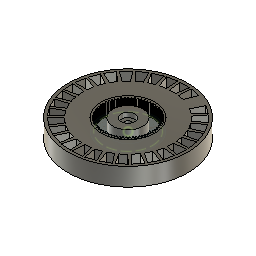
pillbox_disc2 v11 (Autodesk Fusion 360 design; units mm, degrees)
description: Internal Gear; Module: 1.270000; Number of Teeth: 64; Pressure Angle: 20.000000; Root Fillet Radius: 0.040000; Clearance: 0.000000; Gear Thickness: 2.000000; Outer Diameter: 10.000000;
Autodesk Fusion 360 part; units mm, degrees
(part 1 of 2)
sketch "Sketch1" plane through (0, 0, 0) normal (0, 0, 1) x (1, 0, 0)
  circle A0 centre (0, 0) radius 100
  dimension "d3" = 200
  constraint coincident A0.centre origin
  measures "d3" diameter of A0
extrude "Extrude1" add sketch "Sketch1" along normal blind 30 makes body 1
sketch "Sketch2" plane through (0, 0, 30) normal (0, 0, 1) x (-1, 0, 0)
  circle A0 centre (0, 0) radius 100
  line L0 (8, -95) -> (-8, -95)
  line L1 (-8, -95) -> (-5, -75)
  line L2 (-5, -75) -> (5, -75)
  line L3 (5, -75) -> (8, -95)
  line L4 (11.2871, -94.6657) -> (10.1997, -74.4712)
  line L5 (19.995, -72.4583) -> (26.9596, -91.445)
  line L6 (26.9596, -91.445) -> (11.2871, -94.6657)
  line L7 (10.1997, -74.4712) -> (19.995, -72.4583)
  line L8 (30.1121, -90.4558) -> (24.9819, -70.8936)
  line L9 (34.1715, -66.9501) -> (44.8155, -84.1461)
  line L10 (44.8155, -84.1461) -> (30.1121, -90.4558)
  line L11 (24.9819, -70.8936) -> (34.1715, -66.9501)
  line L12 (47.7044, -82.5427) -> (38.7413, -64.4136)
  line L13 (46.9489, -58.7009) -> (60.8366, -73.4024)
  line L14 (60.8366, -73.4024) -> (47.7044, -82.5427)
  line L15 (38.7413, -64.4136) -> (46.9489, -58.7009)
  line L16 (63.3436, -71.2502) -> (50.9146, -55.2965)
  line L17 (57.8043, -48.0486) -> (74.3671, -59.6535)
  line L18 (74.3671, -59.6535) -> (63.3436, -71.2502)
  line L19 (50.9146, -55.2965) -> (57.8043, -48.0486)
  line L20 (76.3895, -57.0407) -> (61.0035, -43.9155)
  line L21 (66.2931, -35.4291) -> (84.8529, -43.4624)
  line L22 (84.8529, -43.4624) -> (76.3895, -57.0407)
  line L23 (61.0035, -43.9155) -> (66.2931, -35.4291)
  line L24 (86.308, -40.496) -> (68.5949, -30.7367)
  line L25 (72.0679, -21.3591) -> (91.8649, -25.492)
  line L26 (91.8649, -25.492) -> (86.308, -40.496)
  line L27 (68.5949, -30.7367) -> (72.0679, -21.3591)
  line L28 (92.6931, -22.2934) -> (73.378, -16.2994)
  line L29 (74.8923, -6.4147) -> (95.1159, -6.4779)
  line L30 (95.1159, -6.4779) -> (92.6931, -22.2934)
  line L31 (73.378, -16.2994) -> (74.8923, -6.4147)
  line L32 (95.2833, -3.1781) -> (75.157, -1.1949)
  line L33 (74.6505, 8.7923) -> (94.4729, 12.8014)
  line L34 (94.4729, 12.8014) -> (95.2833, -3.1781)
  line L35 (75.157, -1.1949) -> (74.6505, 8.7923)
  line L36 (93.9725, 16.0674) -> (73.859, 13.9586)
  line L37 (71.3525, 23.6393) -> (89.9621, 31.5566)
  line L38 (89.9621, 31.5566) -> (93.9725, 16.0674)
  line L39 (73.859, 13.9586) -> (71.3525, 23.6393)
  line L40 (88.8146, 34.655) -> (69.5373, 28.5405)
  line L41 (65.1334, 37.5186) -> (81.7683, 49.0199)
  line L42 (81.7683, 49.0199) -> (88.8146, 34.655)
  line L43 (69.5373, 28.5405) -> (65.1334, 37.5186)
  line L44 (80.0205, 51.8239) -> (62.3687, 41.9541)
  line L45 (56.2477, 49.8618) -> (70.2268, 64.4763)
  line L46 (70.2268, 64.4763) -> (80.0205, 51.8239)
  line L47 (62.3687, 41.9541) -> (56.2477, 49.8618)
  line L48 (67.9505, 66.871) -> (52.6467, 53.65)
  line L49 (45.0591, 60.1637) -> (55.8103, 77.293)
  line L50 (55.8103, 77.293) -> (67.9505, 66.871)
  line L51 (52.6467, 53.65) -> (45.0591, 60.1637)
  line L52 (53.0985, 79.1805) -> (40.7694, 63.1495)
  line L53 (32.0259, 68.0025) -> (39.1089, 86.9453)
  line L54 (39.1089, 86.9453) -> (53.0985, 79.1805)
  line L55 (40.7694, 63.1495) -> (32.0259, 68.0025)
  line L56 (36.0726, 88.2483) -> (27.2229, 70.0636)
  line L57 (17.6815, 73.0573) -> (20.8064, 93.0381)
  line L58 (20.8064, 93.0381) -> (36.0726, 88.2483)
  line L59 (27.2229, 70.0636) -> (17.6815, 73.0573)
  line L60 (17.5699, 93.7032) -> (12.562, 74.1094)
  line L61 (2.6133, 75.121) -> (1.652, 95.3219)
  line L62 (1.652, 95.3219) -> (17.5699, 93.7032)
  line L63 (12.562, 74.1094) -> (2.6133, 75.121)
  line L64 (-1.652, 95.3219) -> (-2.6133, 75.121)
  line L65 (-12.562, 74.1094) -> (-17.5699, 93.7032)
  line L66 (-17.5699, 93.7032) -> (-1.652, 95.3219)
  line L67 (-2.6133, 75.121) -> (-12.562, 74.1094)
  line L68 (-20.8064, 93.0381) -> (-17.6815, 73.0573)
  line L69 (-27.2229, 70.0636) -> (-36.0726, 88.2483)
  line L70 (-36.0726, 88.2483) -> (-20.8064, 93.0381)
  line L71 (-17.6815, 73.0573) -> (-27.2229, 70.0636)
  line L72 (-39.1089, 86.9453) -> (-32.0259, 68.0025)
  line L73 (-40.7694, 63.1495) -> (-53.0985, 79.1805)
  line L74 (-53.0985, 79.1805) -> (-39.1089, 86.9453)
  line L75 (-32.0259, 68.0025) -> (-40.7694, 63.1495)
  line L76 (-55.8103, 77.293) -> (-45.0591, 60.1637)
  line L77 (-52.6467, 53.65) -> (-67.9505, 66.871)
  line L78 (-67.9505, 66.871) -> (-55.8103, 77.293)
  line L79 (-45.0591, 60.1637) -> (-52.6467, 53.65)
  line L80 (-70.2268, 64.4763) -> (-56.2477, 49.8618)
  line L81 (-62.3687, 41.9541) -> (-80.0205, 51.8239)
  line L82 (-80.0205, 51.8239) -> (-70.2268, 64.4763)
  line L83 (-56.2477, 49.8618) -> (-62.3687, 41.9541)
  line L84 (-81.7683, 49.0199) -> (-65.1334, 37.5186)
  line L85 (-69.5373, 28.5405) -> (-88.8146, 34.655)
  line L86 (-88.8146, 34.655) -> (-81.7683, 49.0199)
  line L87 (-65.1334, 37.5186) -> (-69.5373, 28.5405)
  line L88 (-89.9621, 31.5566) -> (-71.3525, 23.6393)
  line L89 (-73.859, 13.9586) -> (-93.9725, 16.0674)
  line L90 (-93.9725, 16.0674) -> (-89.9621, 31.5566)
  line L91 (-71.3525, 23.6393) -> (-73.859, 13.9586)
  line L92 (-94.4729, 12.8014) -> (-74.6505, 8.7923)
  line L93 (-75.157, -1.1949) -> (-95.2833, -3.1781)
  line L94 (-95.2833, -3.1781) -> (-94.4729, 12.8014)
  line L95 (-74.6505, 8.7923) -> (-75.157, -1.1949)
  line L96 (-95.1159, -6.4779) -> (-74.8923, -6.4147)
  line L97 (-73.378, -16.2994) -> (-92.6931, -22.2934)
  line L98 (-92.6931, -22.2934) -> (-95.1159, -6.4779)
  line L99 (-74.8923, -6.4147) -> (-73.378, -16.2994)
  line L100 (-91.8649, -25.492) -> (-72.0679, -21.3591)
  line L101 (-68.5949, -30.7367) -> (-86.308, -40.496)
  line L102 (-86.308, -40.496) -> (-91.8649, -25.492)
  line L103 (-72.0679, -21.3591) -> (-68.5949, -30.7367)
  line L104 (-84.8529, -43.4624) -> (-66.2931, -35.4291)
  line L105 (-61.0035, -43.9155) -> (-76.3895, -57.0407)
  line L106 (-76.3895, -57.0407) -> (-84.8529, -43.4624)
  line L107 (-66.2931, -35.4291) -> (-61.0035, -43.9155)
  line L108 (-74.3671, -59.6535) -> (-57.8043, -48.0486)
  line L109 (-50.9146, -55.2965) -> (-63.3436, -71.2502)
  line L110 (-63.3436, -71.2502) -> (-74.3671, -59.6535)
  line L111 (-57.8043, -48.0486) -> (-50.9146, -55.2965)
  line L112 (-60.8366, -73.4024) -> (-46.9489, -58.7009)
  line L113 (-38.7413, -64.4136) -> (-47.7044, -82.5427)
  line L114 (-47.7044, -82.5427) -> (-60.8366, -73.4024)
  line L115 (-46.9489, -58.7009) -> (-38.7413, -64.4136)
  line L116 (-44.8155, -84.1461) -> (-34.1715, -66.9501)
  line L117 (-24.9819, -70.8936) -> (-30.1121, -90.4558)
  line L118 (-30.1121, -90.4558) -> (-44.8155, -84.1461)
  line L119 (-34.1715, -66.9501) -> (-24.9819, -70.8936)
  line L120 (-26.9596, -91.445) -> (-19.995, -72.4583)
  line L121 (-10.1997, -74.4712) -> (-11.2871, -94.6657)
  line L122 (-11.2871, -94.6657) -> (-26.9596, -91.445)
  line L123 (-19.995, -72.4583) -> (-10.1997, -74.4712)
  dimension "d7" = 360
  constraint horizontal L0
  constraint parallel L0 L2
extrude "Extrude2" cut sketch "Sketch2" against normal blind 30 contours L0 L1 L2 L3 | L4 L5 L6 L7 | L8 L9 L10 L11 | L12 L13 L14 L15 | L16 L17 L18 L19 | L20 L21 L22 L23 | L24 L25 L26 L27 | L28 L29 L30 L31 | L32 L33 L34 L35 | L36 L37 L38 L39 | L40 L41 L42 L43 | L44 L45 L46 L47 | L48 L49 L50 L51 | L52 L53 L54 L55 | L56 L57 L58 L59 | L60 L61 L62 L63 | L64 L65 L66 L67 | L68 L69 L70 L71 | L72 L73 L74 L75 | L76 L77 L78 L79 | L80 L81 L82 L83 | L84 L85 L86 L87 | L88 L89 L90 L91 | L92 L93 L94 L95 | L96 L97 L98 L99 | L100 L101 L102 L103 | L104 L105 L106 L107 | L108 L109 L110 L111 | L112 L113 L114 L115 | L120 L121 L122 L123 bodies 1
sketch "Sketch3" plane through (0, 0, 30) normal (0, 0, 1) x (-1, 0, 0)
  line L0 (26.9596, -91.445) -> (11.2871, -94.6657)
  line L1 (11.2871, -94.6657) -> (10.1997, -74.4712)
  line L2 (10.1997, -74.4712) -> (19.995, -72.4583)
  line L3 (19.995, -72.4583) -> (26.9596, -91.445)
  line L4 (84.8529, -43.4624) -> (76.3895, -57.0407)
  line L5 (76.3895, -57.0407) -> (61.0035, -43.9155)
  line L6 (61.0035, -43.9155) -> (66.2931, -35.4291)
  line L7 (66.2931, -35.4291) -> (84.8529, -43.4624)
  line L8 (89.9621, 31.5566) -> (93.9725, 16.0674)
  line L9 (93.9725, 16.0674) -> (73.859, 13.9586)
  line L10 (73.859, 13.9586) -> (71.3525, 23.6393)
  line L11 (71.3525, 23.6393) -> (89.9621, 31.5566)
  line L12 (39.1089, 86.9453) -> (53.0985, 79.1805)
  line L13 (53.0985, 79.1805) -> (40.7694, 63.1495)
  line L14 (40.7694, 63.1495) -> (32.0259, 68.0025)
  line L15 (32.0259, 68.0025) -> (39.1089, 86.9453)
  line L16 (-36.0726, 88.2483) -> (-20.8064, 93.0381)
  line L17 (-20.8064, 93.0381) -> (-17.6815, 73.0573)
  line L18 (-17.6815, 73.0573) -> (-27.2229, 70.0636)
  line L19 (-27.2229, 70.0636) -> (-36.0726, 88.2483)
  line L20 (-88.8146, 34.655) -> (-81.7683, 49.0199)
  line L21 (-81.7683, 49.0199) -> (-65.1334, 37.5186)
  line L22 (-65.1334, 37.5186) -> (-69.5373, 28.5405)
  line L23 (-69.5373, 28.5405) -> (-88.8146, 34.655)
  line L24 (-86.308, -40.496) -> (-91.8649, -25.492)
  line L25 (-91.8649, -25.492) -> (-72.0679, -21.3591)
  line L26 (-72.0679, -21.3591) -> (-68.5949, -30.7367)
  line L27 (-68.5949, -30.7367) -> (-86.308, -40.496)
  line L28 (-47.7044, -82.5427) -> (-60.8366, -73.4024)
  line L29 (-60.8366, -73.4024) -> (-46.9489, -58.7009)
  line L30 (-46.9489, -58.7009) -> (-38.7413, -64.4136)
  line L31 (-38.7413, -64.4136) -> (-47.7044, -82.5427)
  line L32 (-92.6931, -22.2934) -> (-95.1159, -6.4779)
  line L33 (-95.1159, -6.4779) -> (-74.8923, -6.4147)
  line L34 (-74.8923, -6.4147) -> (-73.378, -16.2994)
  line L35 (-73.378, -16.2994) -> (-92.6931, -22.2934)
  line L36 (-80.0205, 51.8239) -> (-70.2268, 64.4763)
  line L37 (-70.2268, 64.4763) -> (-56.2477, 49.8618)
  line L38 (-56.2477, 49.8618) -> (-62.3687, 41.9541)
  line L39 (-62.3687, 41.9541) -> (-80.0205, 51.8239)
  line L40 (-17.5699, 93.7032) -> (-1.652, 95.3219)
  line L41 (-1.652, 95.3219) -> (-2.6133, 75.121)
  line L42 (-2.6133, 75.121) -> (-12.562, 74.1094)
  line L43 (-12.562, 74.1094) -> (-17.5699, 93.7032)
  line L44 (55.8103, 77.293) -> (67.9505, 66.871)
  line L45 (67.9505, 66.871) -> (52.6467, 53.65)
  line L46 (52.6467, 53.65) -> (45.0591, 60.1637)
  line L47 (45.0591, 60.1637) -> (55.8103, 77.293)
  line L48 (94.4729, 12.8014) -> (95.2833, -3.1781)
  line L49 (95.2833, -3.1781) -> (75.157, -1.1949)
  line L50 (75.157, -1.1949) -> (74.6505, 8.7923)
  line L51 (74.6505, 8.7923) -> (94.4729, 12.8014)
  line L52 (74.3671, -59.6535) -> (63.3436, -71.2502)
  line L53 (63.3436, -71.2502) -> (50.9146, -55.2965)
  line L54 (50.9146, -55.2965) -> (57.8043, -48.0486)
  line L55 (57.8043, -48.0486) -> (74.3671, -59.6535)
  line L56 (-8, -95) -> (-5, -75)
  line L57 (-5, -75) -> (5, -75)
  line L58 (5, -75) -> (8, -95)
  line L59 (8, -95) -> (-8, -95)
  line L60 (44.8155, -84.1461) -> (30.1121, -90.4558)
  line L61 (30.1121, -90.4558) -> (24.9819, -70.8936)
  line L62 (24.9819, -70.8936) -> (34.1715, -66.9501)
  line L63 (34.1715, -66.9501) -> (44.8155, -84.1461)
  line L64 (91.8649, -25.492) -> (86.308, -40.496)
  line L65 (86.308, -40.496) -> (68.5949, -30.7367)
  line L66 (68.5949, -30.7367) -> (72.0679, -21.3591)
  line L67 (72.0679, -21.3591) -> (91.8649, -25.492)
  line L68 (81.7683, 49.0199) -> (88.8146, 34.655)
  line L69 (88.8146, 34.655) -> (69.5373, 28.5405)
  line L70 (69.5373, 28.5405) -> (65.1334, 37.5186)
  line L71 (65.1334, 37.5186) -> (81.7683, 49.0199)
  line L72 (20.8064, 93.0381) -> (36.0726, 88.2483)
  line L73 (36.0726, 88.2483) -> (27.2229, 70.0636)
  line L74 (27.2229, 70.0636) -> (17.6815, 73.0573)
  line L75 (17.6815, 73.0573) -> (20.8064, 93.0381)
  line L76 (-53.0985, 79.1805) -> (-39.1089, 86.9453)
  line L77 (-39.1089, 86.9453) -> (-32.0259, 68.0025)
  line L78 (-32.0259, 68.0025) -> (-40.7694, 63.1495)
  line L79 (-40.7694, 63.1495) -> (-53.0985, 79.1805)
  line L80 (-93.9725, 16.0674) -> (-89.9621, 31.5566)
  line L81 (-89.9621, 31.5566) -> (-71.3525, 23.6393)
  line L82 (-71.3525, 23.6393) -> (-73.859, 13.9586)
  line L83 (-73.859, 13.9586) -> (-93.9725, 16.0674)
  line L84 (-76.3895, -57.0407) -> (-84.8529, -43.4624)
  line L85 (-84.8529, -43.4624) -> (-66.2931, -35.4291)
  line L86 (-66.2931, -35.4291) -> (-61.0035, -43.9155)
  line L87 (-61.0035, -43.9155) -> (-76.3895, -57.0407)
  line L88 (-63.3436, -71.2502) -> (-74.3671, -59.6535)
  line L89 (-74.3671, -59.6535) -> (-57.8043, -48.0486)
  line L90 (-57.8043, -48.0486) -> (-50.9146, -55.2965)
  line L91 (-50.9146, -55.2965) -> (-63.3436, -71.2502)
  line L92 (-95.2833, -3.1781) -> (-94.4729, 12.8014)
  line L93 (-94.4729, 12.8014) -> (-74.6505, 8.7923)
  line L94 (-74.6505, 8.7923) -> (-75.157, -1.1949)
  line L95 (-75.157, -1.1949) -> (-95.2833, -3.1781)
  line L96 (-67.9505, 66.871) -> (-55.8103, 77.293)
  line L97 (-55.8103, 77.293) -> (-45.0591, 60.1637)
  line L98 (-45.0591, 60.1637) -> (-52.6467, 53.65)
  line L99 (-52.6467, 53.65) -> (-67.9505, 66.871)
  line L100 (1.652, 95.3219) -> (17.5699, 93.7032)
  line L101 (17.5699, 93.7032) -> (12.562, 74.1094)
  line L102 (12.562, 74.1094) -> (2.6133, 75.121)
  line L103 (2.6133, 75.121) -> (1.652, 95.3219)
  line L104 (70.2268, 64.4763) -> (80.0205, 51.8239)
  line L105 (80.0205, 51.8239) -> (62.3687, 41.9541)
  line L106 (62.3687, 41.9541) -> (56.2477, 49.8618)
  line L107 (56.2477, 49.8618) -> (70.2268, 64.4763)
  line L108 (95.1159, -6.4779) -> (92.6931, -22.2934)
  line L109 (92.6931, -22.2934) -> (73.378, -16.2994)
  line L110 (73.378, -16.2994) -> (74.8923, -6.4147)
  line L111 (74.8923, -6.4147) -> (95.1159, -6.4779)
  line L112 (60.8366, -73.4024) -> (47.7044, -82.5427)
  line L113 (47.7044, -82.5427) -> (38.7413, -64.4136)
  line L114 (38.7413, -64.4136) -> (46.9489, -58.7009)
  line L115 (46.9489, -58.7009) -> (60.8366, -73.4024)
  line L116 (-11.2871, -94.6657) -> (-26.9596, -91.445)
  line L117 (-26.9596, -91.445) -> (-19.995, -72.4583)
  line L118 (-19.995, -72.4583) -> (-10.1997, -74.4712)
  line L119 (-10.1997, -74.4712) -> (-11.2871, -94.6657)
  circle A0 centre (0, 0) radius 100
  circle A1 centre (0, 0) radius 45
  circle A2 centre (0, 0) radius 25
  dimension "d12" = 90
  dimension "d14" = 50
  constraint coincident A0.centre A1.centre
  measures "d12" diameter of A1
  measures "d14" diameter of A2
extrude "Extrude3" cut sketch "Sketch3" against normal blind 20 contours A1 bodies 1
sketch "Sketch4" plane through (0, 0, 10) normal (0, 0, 1) x (-1, 0, 0)
  circle A0 centre (0, 0) radius 25
  circle A1 centre (0, 0) radius 45
sketch "Sketch1 (2)" plane through (0, 0, 0) normal (0, 1, 0) x (1, 0, 0) in component "Internal Gear (64 teeth)"
  circle A0 centre (0, 0) radius 50
  arc A1 (39.3082, -2.2055) -> (39.5746, -2.6051) centre (39.7076, -2.2279) ccw
  spline S0 degree 3 poles (39.5746, -2.6051) (39.7103, -2.653) (39.8549, -2.7071) (40.0081, -2.7682) knots 0 0 0 0 1 1 1 1
  spline S1 degree 3 poles (40.0081, -2.7682) (40.5817, -2.9968) (41.2726, -3.3224) (42.058, -3.7832) knots 0 0 0 0 1 1 1 1
  arc A2 (41.9879, -4.4946) -> (42.058, -3.7832) centre (0, 0) ccw
  spline S2 degree 3 poles (41.9879, -4.4946) (41.1277, -4.7933) (40.3866, -4.9779) (39.7794, -5.0902) knots 0 0 0 0 1 1 1 1
  spline S3 degree 3 poles (39.7794, -5.0902) (39.6173, -5.1202) (39.4649, -5.1451) (39.3224, -5.1655) knots 0 0 0 0 1 1 1 1
  arc A3 (39.3224, -5.1655) -> (38.9832, -5.5055) centre (39.3792, -5.5615) ccw
  arc A4 (38.9027, -6.0478) -> (38.9832, -5.5055) centre (0, 0) ccw
  arc A5 (38.9027, -6.0478) -> (39.1286, -6.4716) centre (39.298, -6.1092) ccw
  spline S4 degree 3 poles (39.1286, -6.4716) (39.259, -6.5325) (39.3977, -6.6005) (39.5441, -6.6763) knots 0 0 0 0 1 1 1 1
  spline S5 degree 3 poles (39.5441, -6.6763) (40.0925, -6.9601) (40.7482, -7.3518) (41.4846, -7.8874) knots 0 0 0 0 1 1 1 1
  arc A6 (41.3452, -8.5885) -> (41.4846, -7.8874) centre (0, 0) ccw
  spline S6 degree 3 poles (41.3452, -8.5885) (40.4598, -8.8015) (39.7042, -8.9125) (39.0889, -8.9648) knots 0 0 0 0 1 1 1 1
  spline S7 degree 3 poles (39.0889, -8.9648) (38.9246, -8.9788) (38.7705, -8.9885) (38.6267, -8.9949) knots 0 0 0 0 1 1 1 1
  arc A7 (38.6267, -8.9949) -> (38.2558, -9.3) centre (38.6445, -9.3945) ccw
  arc A8 (38.1226, -9.8318) -> (38.2558, -9.3) centre (0, 0) ccw
  arc A9 (38.1226, -9.8318) -> (38.3059, -10.2757) centre (38.5099, -9.9317) ccw
  spline S8 degree 3 poles (38.3059, -10.2757) (38.4297, -10.3491) (38.561, -10.4304) (38.6993, -10.5202) knots 0 0 0 0 1 1 1 1
  spline S9 degree 3 poles (38.6993, -10.5202) (39.2173, -10.8563) (39.8314, -11.3105) (40.5118, -11.9156) knots 0 0 0 0 1 1 1 1
  arc A10 (40.3043, -12.5997) -> (40.5118, -11.9156) centre (0, 0) ccw
  spline S10 degree 3 poles (40.3043, -12.5997) (39.4023, -12.7248) (38.6394, -12.7612) (38.022, -12.753) knots 0 0 0 0 1 1 1 1
  spline S11 degree 3 poles (38.022, -12.753) (37.8571, -12.7508) (37.7028, -12.7454) (37.5591, -12.7377) knots 0 0 0 0 1 1 1 1
  arc A11 (37.5591, -12.7377) -> (37.16, -13.005) centre (37.5376, -13.1371) ccw
  arc A12 (36.9754, -13.5211) -> (37.16, -13.005) centre (0, 0) ccw
  arc A13 (36.9754, -13.5211) -> (37.1143, -13.9809) centre (37.351, -13.6585) ccw
  spline S12 degree 3 poles (37.1143, -13.9809) (37.2303, -14.0661) (37.353, -14.1598) (37.4818, -14.2627) knots 0 0 0 0 1 1 1 1
  spline S13 degree 3 poles (37.4818, -14.2627) (37.9643, -14.648) (38.531, -15.1601) (39.1488, -15.8291) knots 0 0 0 0 1 1 1 1
  arc A14 (38.8752, -16.4895) -> (39.1488, -15.8291) centre (0, 0) ccw
  spline S14 degree 3 poles (38.8752, -16.4895) (37.9653, -16.5257) (37.2025, -16.4871) (36.5889, -16.4184) knots 0 0 0 0 1 1 1 1
  spline S15 degree 3 poles (36.5889, -16.4184) (36.425, -16.4) (36.272, -16.3796) (36.1297, -16.3578) knots 0 0 0 0 1 1 1 1
  arc A15 (36.1297, -16.3578) -> (35.7064, -16.5847) centre (36.0692, -16.7532) ccw
  arc A16 (35.472, -17.0802) -> (35.7064, -16.5847) centre (0, 0) ccw
  arc A17 (35.472, -17.0802) -> (35.5652, -17.5514) centre (35.8324, -17.2537) ccw
  spline S16 degree 3 poles (35.5652, -17.5514) (35.6723, -17.6475) (35.7852, -17.7528) (35.9033, -17.8679) knots 0 0 0 0 1 1 1 1
  spline S17 degree 3 poles (35.9033, -17.8679) (36.3458, -18.2986) (36.8595, -18.8638) (37.4087, -19.5901) knots 0 0 0 0 1 1 1 1
  arc A18 (37.0718, -20.2205) -> (37.4087, -19.5901) centre (0, 0) ccw
  spline S18 degree 3 poles (37.0718, -20.2205) (36.1627, -20.1673) (35.4074, -20.0542) (34.8034, -19.9257) knots 0 0 0 0 1 1 1 1
  spline S19 degree 3 poles (34.8034, -19.9257) (34.6421, -19.8914) (34.4918, -19.856) (34.3524, -19.8203) knots 0 0 0 0 1 1 1 1
  arc A19 (34.3524, -19.8203) -> (33.9089, -20.0046) centre (34.2534, -20.2079) ccw
  arc A20 (33.6271, -20.4748) -> (33.9089, -20.0046) centre (0, 0) ccw
  arc A21 (33.6271, -20.4748) -> (33.6736, -20.9528) centre (33.9687, -20.6829) ccw
  spline S20 degree 3 poles (33.6736, -20.9528) (33.7707, -21.0591) (33.8728, -21.1749) (33.9791, -21.301) knots 0 0 0 0 1 1 1 1
  spline S21 degree 3 poles (33.9791, -21.301) (34.3772, -21.773) (34.833, -22.3859) (35.3084, -23.1625) knots 0 0 0 0 1 1 1 1
  arc A22 (34.9113, -23.7568) -> (35.3084, -23.1625) centre (0, 0) ccw
  spline S22 degree 3 poles (34.9113, -23.7568) (34.0119, -23.6148) (33.2712, -23.4282) (32.6828, -23.2411) knots 0 0 0 0 1 1 1 1
  spline S23 degree 3 poles (32.6828, -23.2411) (32.5256, -23.1911) (32.3795, -23.1411) (32.2442, -23.092) knots 0 0 0 0 1 1 1 1
  arc A23 (32.2442, -23.092) -> (31.7848, -23.232) centre (32.1077, -23.468) ccw
  arc A24 (31.4583, -23.6723) -> (31.7848, -23.232) centre (0, 0) ccw
  arc A25 (31.4583, -23.6723) -> (31.4577, -24.1525) centre (31.7779, -23.9128) ccw
  spline S24 degree 3 poles (31.4577, -24.1525) (31.544, -24.2678) (31.6342, -24.3931) (31.7276, -24.529) knots 0 0 0 0 1 1 1 1
  spline S25 degree 3 poles (31.7276, -24.529) (32.0775, -25.0377) (32.4711, -25.6923) (32.8681, -26.5118) knots 0 0 0 0 1 1 1 1
  arc A26 (32.4146, -27.0644) -> (32.8681, -26.5118) centre (0, 0) ccw
  spline S26 degree 3 poles (32.4146, -27.0644) (31.5334, -26.8348) (30.8146, -26.5765) (30.2474, -26.3326) knots 0 0 0 0 1 1 1 1
  spline S27 degree 3 poles (30.2474, -26.3326) (30.0959, -26.2675) (29.9554, -26.2035) (29.8255, -26.1413) knots 0 0 0 0 1 1 1 1
  arc A27 (29.8255, -26.1413) -> (29.3546, -26.2356) centre (29.6529, -26.5021) ccw
  arc A28 (28.9865, -26.6417) -> (29.3546, -26.2356) centre (0, 0) ccw
  arc A29 (28.9865, -26.6417) -> (28.9389, -27.1196) centre (29.281, -26.9124) ccw
  spline S28 degree 3 poles (28.9389, -27.1196) (29.0134, -27.2428) (29.0909, -27.3763) (29.1706, -27.5207) knots 0 0 0 0 1 1 1 1
  spline S29 degree 3 poles (29.1706, -27.5207) (29.4689, -28.0613) (29.7964, -28.7513) (30.1112, -29.6058) knots 0 0 0 0 1 1 1 1
  arc A30 (29.6058, -30.1112) -> (30.1112, -29.6058) centre (0, 0) ccw
  spline S30 degree 3 poles (29.6058, -30.1112) (28.7513, -29.7964) (28.0613, -29.4689) (27.5207, -29.1706) knots 0 0 0 0 1 1 1 1
  spline S31 degree 3 poles (27.5207, -29.1706) (27.3763, -29.0909) (27.2428, -29.0134) (27.1196, -28.9389) knots 0 0 0 0 1 1 1 1
  arc A31 (27.1196, -28.9389) -> (26.6417, -28.9865) centre (26.9124, -29.281) ccw
  arc A32 (26.2356, -29.3546) -> (26.6417, -28.9865) centre (0, 0) ccw
  arc A33 (26.2356, -29.3546) -> (26.1413, -29.8255) centre (26.5021, -29.6529) ccw
  spline S32 degree 3 poles (26.1413, -29.8255) (26.2035, -29.9554) (26.2675, -30.0959) (26.3326, -30.2474) knots 0 0 0 0 1 1 1 1
  spline S33 degree 3 poles (26.3326, -30.2474) (26.5765, -30.8146) (26.8348, -31.5334) (27.0644, -32.4146) knots 0 0 0 0 1 1 1 1
  arc A34 (26.5118, -32.8681) -> (27.0644, -32.4146) centre (0, 0) ccw
  spline S34 degree 3 poles (26.5118, -32.8681) (25.6923, -32.4711) (25.0377, -32.0775) (24.529, -31.7276) knots 0 0 0 0 1 1 1 1
  spline S35 degree 3 poles (24.529, -31.7276) (24.3931, -31.6342) (24.2678, -31.544) (24.1525, -31.4577) knots 0 0 0 0 1 1 1 1
  arc A35 (24.1525, -31.4577) -> (23.6723, -31.4583) centre (23.9128, -31.7779) ccw
  arc A36 (23.232, -31.7848) -> (23.6723, -31.4583) centre (0, 0) ccw
  arc A37 (23.232, -31.7848) -> (23.092, -32.2442) centre (23.468, -32.1077) ccw
  spline S36 degree 3 poles (23.092, -32.2442) (23.1411, -32.3795) (23.1911, -32.5256) (23.2411, -32.6828) knots 0 0 0 0 1 1 1 1
  spline S37 degree 3 poles (23.2411, -32.6828) (23.4282, -33.2712) (23.6148, -34.0119) (23.7568, -34.9113) knots 0 0 0 0 1 1 1 1
  arc A38 (23.1625, -35.3084) -> (23.7568, -34.9113) centre (0, 0) ccw
  spline S38 degree 3 poles (23.1625, -35.3084) (22.3859, -34.833) (21.773, -34.3772) (21.301, -33.9791) knots 0 0 0 0 1 1 1 1
  spline S39 degree 3 poles (21.301, -33.9791) (21.1749, -33.8728) (21.0591, -33.7707) (20.9528, -33.6736) knots 0 0 0 0 1 1 1 1
  arc A39 (20.9528, -33.6736) -> (20.4748, -33.6271) centre (20.6829, -33.9687) ccw
  arc A40 (20.0046, -33.9089) -> (20.4748, -33.6271) centre (0, 0) ccw
  arc A41 (20.0046, -33.9089) -> (19.8203, -34.3524) centre (20.2079, -34.2534) ccw
  spline S40 degree 3 poles (19.8203, -34.3524) (19.856, -34.4918) (19.8914, -34.6421) (19.9257, -34.8034) knots 0 0 0 0 1 1 1 1
  spline S41 degree 3 poles (19.9257, -34.8034) (20.0542, -35.4074) (20.1673, -36.1627) (20.2205, -37.0718) knots 0 0 0 0 1 1 1 1
  arc A42 (19.5901, -37.4087) -> (20.2205, -37.0718) centre (0, 0) ccw
  spline S42 degree 3 poles (19.5901, -37.4087) (18.8638, -36.8595) (18.2986, -36.3458) (17.8679, -35.9033) knots 0 0 0 0 1 1 1 1
  spline S43 degree 3 poles (17.8679, -35.9033) (17.7528, -35.7852) (17.6475, -35.6723) (17.5514, -35.5652) knots 0 0 0 0 1 1 1 1
  arc A43 (17.5514, -35.5652) -> (17.0802, -35.472) centre (17.2537, -35.8324) ccw
  arc A44 (16.5847, -35.7064) -> (17.0802, -35.472) centre (0, 0) ccw
  arc A45 (16.5847, -35.7064) -> (16.3578, -36.1297) centre (16.7532, -36.0692) ccw
  spline S44 degree 3 poles (16.3578, -36.1297) (16.3796, -36.272) (16.4, -36.425) (16.4184, -36.5889) knots 0 0 0 0 1 1 1 1
  spline S45 degree 3 poles (16.4184, -36.5889) (16.4871, -37.2025) (16.5257, -37.9653) (16.4895, -38.8752) knots 0 0 0 0 1 1 1 1
  arc A46 (15.8291, -39.1488) -> (16.4895, -38.8752) centre (0, 0) ccw
  spline S46 degree 3 poles (15.8291, -39.1488) (15.1601, -38.531) (14.648, -37.9643) (14.2627, -37.4818) knots 0 0 0 0 1 1 1 1
  spline S47 degree 3 poles (14.2627, -37.4818) (14.1598, -37.353) (14.0661, -37.2303) (13.9809, -37.1143) knots 0 0 0 0 1 1 1 1
  arc A47 (13.9809, -37.1143) -> (13.5211, -36.9754) centre (13.6585, -37.351) ccw
  arc A48 (13.005, -37.16) -> (13.5211, -36.9754) centre (0, 0) ccw
  arc A49 (13.005, -37.16) -> (12.7377, -37.5591) centre (13.1371, -37.5376) ccw
  spline S48 degree 3 poles (12.7377, -37.5591) (12.7454, -37.7028) (12.7508, -37.8571) (12.753, -38.022) knots 0 0 0 0 1 1 1 1
  spline S49 degree 3 poles (12.753, -38.022) (12.7612, -38.6394) (12.7248, -39.4023) (12.5997, -40.3043) knots 0 0 0 0 1 1 1 1
  arc A50 (11.9156, -40.5118) -> (12.5997, -40.3043) centre (0, 0) ccw
  spline S50 degree 3 poles (11.9156, -40.5118) (11.3105, -39.8314) (10.8563, -39.2173) (10.5202, -38.6993) knots 0 0 0 0 1 1 1 1
  spline S51 degree 3 poles (10.5202, -38.6993) (10.4304, -38.561) (10.3491, -38.4297) (10.2757, -38.3059) knots 0 0 0 0 1 1 1 1
  arc A51 (10.2757, -38.3059) -> (9.8318, -38.1226) centre (9.9317, -38.5099) ccw
  arc A52 (9.3, -38.2558) -> (9.8318, -38.1226) centre (0, 0) ccw
  arc A53 (9.3, -38.2558) -> (8.9949, -38.6267) centre (9.3945, -38.6445) ccw
  spline S52 degree 3 poles (8.9949, -38.6267) (8.9885, -38.7705) (8.9788, -38.9246) (8.9648, -39.0889) knots 0 0 0 0 1 1 1 1
  spline S53 degree 3 poles (8.9648, -39.0889) (8.9125, -39.7042) (8.8015, -40.4598) (8.5885, -41.3452) knots 0 0 0 0 1 1 1 1
  arc A54 (7.8874, -41.4846) -> (8.5885, -41.3452) centre (0, 0) ccw
  spline S54 degree 3 poles (7.8874, -41.4846) (7.3518, -40.7482) (6.9601, -40.0925) (6.6763, -39.5441) knots 0 0 0 0 1 1 1 1
  spline S55 degree 3 poles (6.6763, -39.5441) (6.6005, -39.3977) (6.5325, -39.259) (6.4716, -39.1286) knots 0 0 0 0 1 1 1 1
  arc A55 (6.4716, -39.1286) -> (6.0478, -38.9027) centre (6.1092, -39.298) ccw
  arc A56 (5.5055, -38.9832) -> (6.0478, -38.9027) centre (0, 0) ccw
  arc A57 (5.5055, -38.9832) -> (5.1655, -39.3224) centre (5.5615, -39.3792) ccw
  spline S56 degree 3 poles (5.1655, -39.3224) (5.1451, -39.4649) (5.1202, -39.6173) (5.0902, -39.7794) knots 0 0 0 0 1 1 1 1
  spline S57 degree 3 poles (5.0902, -39.7794) (4.9779, -40.3866) (4.7933, -41.1277) (4.4946, -41.9879) knots 0 0 0 0 1 1 1 1
  arc A58 (3.7832, -42.058) -> (4.4946, -41.9879) centre (0, 0) ccw
  spline S58 degree 3 poles (3.7832, -42.058) (3.3224, -41.2726) (2.9968, -40.5817) (2.7682, -40.0081) knots 0 0 0 0 1 1 1 1
  spline S59 degree 3 poles (2.7682, -40.0081) (2.7071, -39.8549) (2.653, -39.7103) (2.6051, -39.5746) knots 0 0 0 0 1 1 1 1
  arc A59 (2.6051, -39.5746) -> (2.2055, -39.3082) centre (2.2279, -39.7076) ccw
  arc A60 (1.658, -39.3351) -> (2.2055, -39.3082) centre (0, 0) ccw
  arc A61 (1.658, -39.3351) -> (1.2864, -39.6393) centre (1.6748, -39.7347) ccw
  spline S60 degree 3 poles (1.2864, -39.6393) (1.2521, -39.7791) (1.2124, -39.9284) (1.1666, -40.0868) knots 0 0 0 0 1 1 1 1
  spline S61 degree 3 poles (1.1666, -40.0868) (0.9953, -40.68) (0.739, -41.3995) (0.3574, -42.2263) knots 0 0 0 0 1 1 1 1
  arc A62 (-0.3574, -42.2263) -> (0.3574, -42.2263) centre (0, 0) ccw
  spline S62 degree 3 poles (-0.3574, -42.2263) (-0.739, -41.3995) (-0.9953, -40.68) (-1.1666, -40.0868) knots 0 0 0 0 1 1 1 1
  spline S63 degree 3 poles (-1.1666, -40.0868) (-1.2124, -39.9284) (-1.2521, -39.7791) (-1.2864, -39.6393) knots 0 0 0 0 1 1 1 1
  arc A63 (-1.2864, -39.6393) -> (-1.658, -39.3351) centre (-1.6748, -39.7347) ccw
  arc A64 (-2.2055, -39.3082) -> (-1.658, -39.3351) centre (0, 0) ccw
  arc A65 (-2.2055, -39.3082) -> (-2.6051, -39.5746) centre (-2.2279, -39.7076) ccw
  spline S64 degree 3 poles (-2.6051, -39.5746) (-2.653, -39.7103) (-2.7071, -39.8549) (-2.7682, -40.0081) knots 0 0 0 0 1 1 1 1
  spline S65 degree 3 poles (-2.7682, -40.0081) (-2.9968, -40.5817) (-3.3224, -41.2726) (-3.7832, -42.058) knots 0 0 0 0 1 1 1 1
  arc A66 (-4.4946, -41.9879) -> (-3.7832, -42.058) centre (0, 0) ccw
  spline S66 degree 3 poles (-4.4946, -41.9879) (-4.7933, -41.1277) (-4.9779, -40.3866) (-5.0902, -39.7794) knots 0 0 0 0 1 1 1 1
  spline S67 degree 3 poles (-5.0902, -39.7794) (-5.1202, -39.6173) (-5.1451, -39.4649) (-5.1655, -39.3224) knots 0 0 0 0 1 1 1 1
  arc A67 (-5.1655, -39.3224) -> (-5.5055, -38.9832) centre (-5.5615, -39.3792) ccw
  arc A68 (-6.0478, -38.9027) -> (-5.5055, -38.9832) centre (0, 0) ccw
  arc A69 (-6.0478, -38.9027) -> (-6.4716, -39.1286) centre (-6.1092, -39.298) ccw
  spline S68 degree 3 poles (-6.4716, -39.1286) (-6.5325, -39.259) (-6.6005, -39.3977) (-6.6763, -39.5441) knots 0 0 0 0 1 1 1 1
  spline S69 degree 3 poles (-6.6763, -39.5441) (-6.9601, -40.0925) (-7.3518, -40.7482) (-7.8874, -41.4846) knots 0 0 0 0 1 1 1 1
  arc A70 (-8.5885, -41.3452) -> (-7.8874, -41.4846) centre (0, 0) ccw
  spline S70 degree 3 poles (-8.5885, -41.3452) (-8.8015, -40.4598) (-8.9125, -39.7042) (-8.9648, -39.0889) knots 0 0 0 0 1 1 1 1
  spline S71 degree 3 poles (-8.9648, -39.0889) (-8.9788, -38.9246) (-8.9885, -38.7705) (-8.9949, -38.6267) knots 0 0 0 0 1 1 1 1
  arc A71 (-8.9949, -38.6267) -> (-9.3, -38.2558) centre (-9.3945, -38.6445) ccw
  arc A72 (-9.8318, -38.1226) -> (-9.3, -38.2558) centre (0, 0) ccw
  arc A73 (-9.8318, -38.1226) -> (-10.2757, -38.3059) centre (-9.9317, -38.5099) ccw
  spline S72 degree 3 poles (-10.2757, -38.3059) (-10.3491, -38.4297) (-10.4304, -38.561) (-10.5202, -38.6993) knots 0 0 0 0 1 1 1 1
  spline S73 degree 3 poles (-10.5202, -38.6993) (-10.8563, -39.2173) (-11.3105, -39.8314) (-11.9156, -40.5118) knots 0 0 0 0 1 1 1 1
  arc A74 (-12.5997, -40.3043) -> (-11.9156, -40.5118) centre (0, 0) ccw
  spline S74 degree 3 poles (-12.5997, -40.3043) (-12.7248, -39.4023) (-12.7612, -38.6394) (-12.753, -38.022) knots 0 0 0 0 1 1 1 1
  spline S75 degree 3 poles (-12.753, -38.022) (-12.7508, -37.8571) (-12.7454, -37.7028) (-12.7377, -37.5591) knots 0 0 0 0 1 1 1 1
  arc A75 (-12.7377, -37.5591) -> (-13.005, -37.16) centre (-13.1371, -37.5376) ccw
  arc A76 (-13.5211, -36.9754) -> (-13.005, -37.16) centre (0, 0) ccw
  arc A77 (-13.5211, -36.9754) -> (-13.9809, -37.1143) centre (-13.6585, -37.351) ccw
  spline S76 degree 3 poles (-13.9809, -37.1143) (-14.0661, -37.2303) (-14.1598, -37.353) (-14.2627, -37.4818) knots 0 0 0 0 1 1 1 1
  spline S77 degree 3 poles (-14.2627, -37.4818) (-14.648, -37.9643) (-15.1601, -38.531) (-15.8291, -39.1488) knots 0 0 0 0 1 1 1 1
  arc A78 (-16.4895, -38.8752) -> (-15.8291, -39.1488) centre (0, 0) ccw
  spline S78 degree 3 poles (-16.4895, -38.8752) (-16.5257, -37.9653) (-16.4871, -37.2025) (-16.4184, -36.5889) knots 0 0 0 0 1 1 1 1
  spline S79 degree 3 poles (-16.4184, -36.5889) (-16.4, -36.425) (-16.3796, -36.272) (-16.3578, -36.1297) knots 0 0 0 0 1 1 1 1
  arc A79 (-16.3578, -36.1297) -> (-16.5847, -35.7064) centre (-16.7532, -36.0692) ccw
  arc A80 (-17.0802, -35.472) -> (-16.5847, -35.7064) centre (0, 0) ccw
  arc A81 (-17.0802, -35.472) -> (-17.5514, -35.5652) centre (-17.2537, -35.8324) ccw
  spline S80 degree 3 poles (-17.5514, -35.5652) (-17.6475, -35.6723) (-17.7528, -35.7852) (-17.8679, -35.9033) knots 0 0 0 0 1 1 1 1
  spline S81 degree 3 poles (-17.8679, -35.9033) (-18.2986, -36.3458) (-18.8638, -36.8595) (-19.5901, -37.4087) knots 0 0 0 0 1 1 1 1
  arc A82 (-20.2205, -37.0718) -> (-19.5901, -37.4087) centre (0, 0) ccw
  spline S82 degree 3 poles (-20.2205, -37.0718) (-20.1673, -36.1627) (-20.0542, -35.4074) (-19.9257, -34.8034) knots 0 0 0 0 1 1 1 1
  spline S83 degree 3 poles (-19.9257, -34.8034) (-19.8914, -34.6421) (-19.856, -34.4918) (-19.8203, -34.3524) knots 0 0 0 0 1 1 1 1
  arc A83 (-19.8203, -34.3524) -> (-20.0046, -33.9089) centre (-20.2079, -34.2534) ccw
  arc A84 (-20.4748, -33.6271) -> (-20.0046, -33.9089) centre (0, 0) ccw
  arc A85 (-20.4748, -33.6271) -> (-20.9528, -33.6736) centre (-20.6829, -33.9687) ccw
  spline S84 degree 3 poles (-20.9528, -33.6736) (-21.0591, -33.7707) (-21.1749, -33.8728) (-21.301, -33.9791) knots 0 0 0 0 1 1 1 1
  spline S85 degree 3 poles (-21.301, -33.9791) (-21.773, -34.3772) (-22.3859, -34.833) (-23.1625, -35.3084) knots 0 0 0 0 1 1 1 1
  arc A86 (-23.7568, -34.9113) -> (-23.1625, -35.3084) centre (0, 0) ccw
  spline S86 degree 3 poles (-23.7568, -34.9113) (-23.6148, -34.0119) (-23.4282, -33.2712) (-23.2411, -32.6828) knots 0 0 0 0 1 1 1 1
  spline S87 degree 3 poles (-23.2411, -32.6828) (-23.1911, -32.5256) (-23.1411, -32.3795) (-23.092, -32.2442) knots 0 0 0 0 1 1 1 1
  arc A87 (-23.092, -32.2442) -> (-23.232, -31.7848) centre (-23.468, -32.1077) ccw
  arc A88 (-23.6723, -31.4583) -> (-23.232, -31.7848) centre (0, 0) ccw
  arc A89 (-23.6723, -31.4583) -> (-24.1525, -31.4577) centre (-23.9128, -31.7779) ccw
  spline S88 degree 3 poles (-24.1525, -31.4577) (-24.2678, -31.544) (-24.3931, -31.6342) (-24.529, -31.7276) knots 0 0 0 0 1 1 1 1
  spline S89 degree 3 poles (-24.529, -31.7276) (-25.0377, -32.0775) (-25.6923, -32.4711) (-26.5118, -32.8681) knots 0 0 0 0 1 1 1 1
  arc A90 (-27.0644, -32.4146) -> (-26.5118, -32.8681) centre (0, 0) ccw
  spline S90 degree 3 poles (-27.0644, -32.4146) (-26.8348, -31.5334) (-26.5765, -30.8146) (-26.3326, -30.2474) knots 0 0 0 0 1 1 1 1
  spline S91 degree 3 poles (-26.3326, -30.2474) (-26.2675, -30.0959) (-26.2035, -29.9554) (-26.1413, -29.8255) knots 0 0 0 0 1 1 1 1
  arc A91 (-26.1413, -29.8255) -> (-26.2356, -29.3546) centre (-26.5021, -29.6529) ccw
  arc A92 (-26.6417, -28.9865) -> (-26.2356, -29.3546) centre (0, 0) ccw
  arc A93 (-26.6417, -28.9865) -> (-27.1196, -28.9389) centre (-26.9124, -29.281) ccw
  spline S92 degree 3 poles (-27.1196, -28.9389) (-27.2428, -29.0134) (-27.3763, -29.0909) (-27.5207, -29.1706) knots 0 0 0 0 1 1 1 1
  spline S93 degree 3 poles (-27.5207, -29.1706) (-28.0613, -29.4689) (-28.7513, -29.7964) (-29.6058, -30.1112) knots 0 0 0 0 1 1 1 1
  arc A94 (-30.1112, -29.6058) -> (-29.6058, -30.1112) centre (0, 0) ccw
  spline S94 degree 3 poles (-30.1112, -29.6058) (-29.7964, -28.7513) (-29.4689, -28.0613) (-29.1706, -27.5207) knots 0 0 0 0 1 1 1 1
  spline S95 degree 3 poles (-29.1706, -27.5207) (-29.0909, -27.3763) (-29.0134, -27.2428) (-28.9389, -27.1196) knots 0 0 0 0 1 1 1 1
  arc A95 (-28.9389, -27.1196) -> (-28.9865, -26.6417) centre (-29.281, -26.9124) ccw
  arc A96 (-29.3546, -26.2356) -> (-28.9865, -26.6417) centre (0, 0) ccw
  arc A97 (-29.3546, -26.2356) -> (-29.8255, -26.1413) centre (-29.6529, -26.5021) ccw
  spline S96 degree 3 poles (-29.8255, -26.1413) (-29.9554, -26.2035) (-30.0959, -26.2675) (-30.2474, -26.3326) knots 0 0 0 0 1 1 1 1
  spline S97 degree 3 poles (-30.2474, -26.3326) (-30.8146, -26.5765) (-31.5334, -26.8348) (-32.4146, -27.0644) knots 0 0 0 0 1 1 1 1
  arc A98 (-32.8681, -26.5118) -> (-32.4146, -27.0644) centre (0, 0) ccw
  spline S98 degree 3 poles (-32.8681, -26.5118) (-32.4711, -25.6923) (-32.0775, -25.0377) (-31.7276, -24.529) knots 0 0 0 0 1 1 1 1
  spline S99 degree 3 poles (-31.7276, -24.529) (-31.6342, -24.3931) (-31.544, -24.2678) (-31.4577, -24.1525) knots 0 0 0 0 1 1 1 1
  arc A99 (-31.4577, -24.1525) -> (-31.4583, -23.6723) centre (-31.7779, -23.9128) ccw
  arc A100 (-31.7848, -23.232) -> (-31.4583, -23.6723) centre (0, 0) ccw
  arc A101 (-31.7848, -23.232) -> (-32.2442, -23.092) centre (-32.1077, -23.468) ccw
  spline S100 degree 3 poles (-32.2442, -23.092) (-32.3795, -23.1411) (-32.5256, -23.1911) (-32.6828, -23.2411) knots 0 0 0 0 1 1 1 1
  spline S101 degree 3 poles (-32.6828, -23.2411) (-33.2712, -23.4282) (-34.0119, -23.6148) (-34.9113, -23.7568) knots 0 0 0 0 1 1 1 1
  arc A102 (-35.3084, -23.1625) -> (-34.9113, -23.7568) centre (0, 0) ccw
  spline S102 degree 3 poles (-35.3084, -23.1625) (-34.833, -22.3859) (-34.3772, -21.773) (-33.9791, -21.301) knots 0 0 0 0 1 1 1 1
  spline S103 degree 3 poles (-33.9791, -21.301) (-33.8728, -21.1749) (-33.7707, -21.0591) (-33.6736, -20.9528) knots 0 0 0 0 1 1 1 1
  arc A103 (-33.6736, -20.9528) -> (-33.6271, -20.4748) centre (-33.9687, -20.6829) ccw
  arc A104 (-33.9089, -20.0046) -> (-33.6271, -20.4748) centre (0, 0) ccw
  arc A105 (-33.9089, -20.0046) -> (-34.3524, -19.8203) centre (-34.2534, -20.2079) ccw
  spline S104 degree 3 poles (-34.3524, -19.8203) (-34.4918, -19.856) (-34.6421, -19.8914) (-34.8034, -19.9257) knots 0 0 0 0 1 1 1 1
  spline S105 degree 3 poles (-34.8034, -19.9257) (-35.4074, -20.0542) (-36.1627, -20.1673) (-37.0718, -20.2205) knots 0 0 0 0 1 1 1 1
  arc A106 (-37.4087, -19.5901) -> (-37.0718, -20.2205) centre (0, 0) ccw
  spline S106 degree 3 poles (-37.4087, -19.5901) (-36.8595, -18.8638) (-36.3458, -18.2986) (-35.9033, -17.8679) knots 0 0 0 0 1 1 1 1
  spline S107 degree 3 poles (-35.9033, -17.8679) (-35.7852, -17.7528) (-35.6723, -17.6475) (-35.5652, -17.5514) knots 0 0 0 0 1 1 1 1
  arc A107 (-35.5652, -17.5514) -> (-35.472, -17.0802) centre (-35.8324, -17.2537) ccw
  arc A108 (-35.7064, -16.5847) -> (-35.472, -17.0802) centre (0, 0) ccw
  arc A109 (-35.7064, -16.5847) -> (-36.1297, -16.3578) centre (-36.0692, -16.7532) ccw
  spline S108 degree 3 poles (-36.1297, -16.3578) (-36.272, -16.3796) (-36.425, -16.4) (-36.5889, -16.4184) knots 0 0 0 0 1 1 1 1
  spline S109 degree 3 poles (-36.5889, -16.4184) (-37.2025, -16.4871) (-37.9653, -16.5257) (-38.8752, -16.4895) knots 0 0 0 0 1 1 1 1
  arc A110 (-39.1488, -15.8291) -> (-38.8752, -16.4895) centre (0, 0) ccw
  spline S110 degree 3 poles (-39.1488, -15.8291) (-38.531, -15.1601) (-37.9643, -14.648) (-37.4818, -14.2627) knots 0 0 0 0 1 1 1 1
  spline S111 degree 3 poles (-37.4818, -14.2627) (-37.353, -14.1598) (-37.2303, -14.0661) (-37.1143, -13.9809) knots 0 0 0 0 1 1 1 1
  arc A111 (-37.1143, -13.9809) -> (-36.9754, -13.5211) centre (-37.351, -13.6585) ccw
  arc A112 (-37.16, -13.005) -> (-36.9754, -13.5211) centre (0, 0) ccw
  arc A113 (-37.16, -13.005) -> (-37.5591, -12.7377) centre (-37.5376, -13.1371) ccw
  spline S112 degree 3 poles (-37.5591, -12.7377) (-37.7028, -12.7454) (-37.8571, -12.7508) (-38.022, -12.753) knots 0 0 0 0 1 1 1 1
  spline S113 degree 3 poles (-38.022, -12.753) (-38.6394, -12.7612) (-39.4023, -12.7248) (-40.3043, -12.5997) knots 0 0 0 0 1 1 1 1
  arc A114 (-40.5118, -11.9156) -> (-40.3043, -12.5997) centre (0, 0) ccw
  spline S114 degree 3 poles (-40.5118, -11.9156) (-39.8314, -11.3105) (-39.2173, -10.8563) (-38.6993, -10.5202) knots 0 0 0 0 1 1 1 1
  spline S115 degree 3 poles (-38.6993, -10.5202) (-38.561, -10.4304) (-38.4297, -10.3491) (-38.3059, -10.2757) knots 0 0 0 0 1 1 1 1
  arc A115 (-38.3059, -10.2757) -> (-38.1226, -9.8318) centre (-38.5099, -9.9317) ccw
  arc A116 (-38.2558, -9.3) -> (-38.1226, -9.8318) centre (0, 0) ccw
  arc A117 (-38.2558, -9.3) -> (-38.6267, -8.9949) centre (-38.6445, -9.3945) ccw
  spline S116 degree 3 poles (-38.6267, -8.9949) (-38.7705, -8.9885) (-38.9246, -8.9788) (-39.0889, -8.9648) knots 0 0 0 0 1 1 1 1
  spline S117 degree 3 poles (-39.0889, -8.9648) (-39.7042, -8.9125) (-40.4598, -8.8015) (-41.3452, -8.5885) knots 0 0 0 0 1 1 1 1
  arc A118 (-41.4846, -7.8874) -> (-41.3452, -8.5885) centre (0, 0) ccw
  spline S118 degree 3 poles (-41.4846, -7.8874) (-40.7482, -7.3518) (-40.0925, -6.9601) (-39.5441, -6.6763) knots 0 0 0 0 1 1 1 1
  spline S119 degree 3 poles (-39.5441, -6.6763) (-39.3977, -6.6005) (-39.259, -6.5325) (-39.1286, -6.4716) knots 0 0 0 0 1 1 1 1
  arc A119 (-39.1286, -6.4716) -> (-38.9027, -6.0478) centre (-39.298, -6.1092) ccw
  arc A120 (-38.9832, -5.5055) -> (-38.9027, -6.0478) centre (0, 0) ccw
  arc A121 (-38.9832, -5.5055) -> (-39.3224, -5.1655) centre (-39.3792, -5.5615) ccw
  spline S120 degree 3 poles (-39.3224, -5.1655) (-39.4649, -5.1451) (-39.6173, -5.1202) (-39.7794, -5.0902) knots 0 0 0 0 1 1 1 1
  spline S121 degree 3 poles (-39.7794, -5.0902) (-40.3866, -4.9779) (-41.1277, -4.7933) (-41.9879, -4.4946) knots 0 0 0 0 1 1 1 1
  arc A122 (-42.058, -3.7832) -> (-41.9879, -4.4946) centre (0, 0) ccw
  spline S122 degree 3 poles (-42.058, -3.7832) (-41.2726, -3.3224) (-40.5817, -2.9968) (-40.0081, -2.7682) knots 0 0 0 0 1 1 1 1
  spline S123 degree 3 poles (-40.0081, -2.7682) (-39.8549, -2.7071) (-39.7103, -2.653) (-39.5746, -2.6051) knots 0 0 0 0 1 1 1 1
  arc A123 (-39.5746, -2.6051) -> (-39.3082, -2.2055) centre (-39.7076, -2.2279) ccw
  arc A124 (-39.3351, -1.658) -> (-39.3082, -2.2055) centre (0, 0) ccw
  arc A125 (-39.3351, -1.658) -> (-39.6393, -1.2864) centre (-39.7347, -1.6748) ccw
  spline S124 degree 3 poles (-39.6393, -1.2864) (-39.7791, -1.2521) (-39.9284, -1.2124) (-40.0868, -1.1666) knots 0 0 0 0 1 1 1 1
  spline S125 degree 3 poles (-40.0868, -1.1666) (-40.68, -0.9953) (-41.3995, -0.739) (-42.2263, -0.3574) knots 0 0 0 0 1 1 1 1
  arc A126 (-42.2263, 0.3574) -> (-42.2263, -0.3574) centre (0, 0) ccw
  spline S126 degree 3 poles (-42.2263, 0.3574) (-41.3995, 0.739) (-40.68, 0.9953) (-40.0868, 1.1666) knots 0 0 0 0 1 1 1 1
  spline S127 degree 3 poles (-40.0868, 1.1666) (-39.9284, 1.2124) (-39.7791, 1.2521) (-39.6393, 1.2864) knots 0 0 0 0 1 1 1 1
  arc A127 (-39.6393, 1.2864) -> (-39.3351, 1.658) centre (-39.7347, 1.6748) ccw
  arc A128 (-39.3082, 2.2055) -> (-39.3351, 1.658) centre (0, 0) ccw
  arc A129 (-39.3082, 2.2055) -> (-39.5746, 2.6051) centre (-39.7076, 2.2279) ccw
  spline S128 degree 3 poles (-39.5746, 2.6051) (-39.7103, 2.653) (-39.8549, 2.7071) (-40.0081, 2.7682) knots 0 0 0 0 1 1 1 1
  spline S129 degree 3 poles (-40.0081, 2.7682) (-40.5817, 2.9968) (-41.2726, 3.3224) (-42.058, 3.7832) knots 0 0 0 0 1 1 1 1
  arc A130 (-41.9879, 4.4946) -> (-42.058, 3.7832) centre (0, 0) ccw
  spline S130 degree 3 poles (-41.9879, 4.4946) (-41.1277, 4.7933) (-40.3866, 4.9779) (-39.7794, 5.0902) knots 0 0 0 0 1 1 1 1
  spline S131 degree 3 poles (-39.7794, 5.0902) (-39.6173, 5.1202) (-39.4649, 5.1451) (-39.3224, 5.1655) knots 0 0 0 0 1 1 1 1
  arc A131 (-39.3224, 5.1655) -> (-38.9832, 5.5055) centre (-39.3792, 5.5615) ccw
  arc A132 (-38.9027, 6.0478) -> (-38.9832, 5.5055) centre (0, 0) ccw
  arc A133 (-38.9027, 6.0478) -> (-39.1286, 6.4716) centre (-39.298, 6.1092) ccw
  spline S132 degree 3 poles (-39.1286, 6.4716) (-39.259, 6.5325) (-39.3977, 6.6005) (-39.5441, 6.6763) knots 0 0 0 0 1 1 1 1
  spline S133 degree 3 poles (-39.5441, 6.6763) (-40.0925, 6.9601) (-40.7482, 7.3518) (-41.4846, 7.8874) knots 0 0 0 0 1 1 1 1
  arc A134 (-41.3452, 8.5885) -> (-41.4846, 7.8874) centre (0, 0) ccw
  spline S134 degree 3 poles (-41.3452, 8.5885) (-40.4598, 8.8015) (-39.7042, 8.9125) (-39.0889, 8.9648) knots 0 0 0 0 1 1 1 1
  spline S135 degree 3 poles (-39.0889, 8.9648) (-38.9246, 8.9788) (-38.7705, 8.9885) (-38.6267, 8.9949) knots 0 0 0 0 1 1 1 1
  arc A135 (-38.6267, 8.9949) -> (-38.2558, 9.3) centre (-38.6445, 9.3945) ccw
  arc A136 (-38.1226, 9.8318) -> (-38.2558, 9.3) centre (0, 0) ccw
  arc A137 (-38.1226, 9.8318) -> (-38.3059, 10.2757) centre (-38.5099, 9.9317) ccw
  spline S136 degree 3 poles (-38.3059, 10.2757) (-38.4297, 10.3491) (-38.561, 10.4304) (-38.6993, 10.5202) knots 0 0 0 0 1 1 1 1
  spline S137 degree 3 poles (-38.6993, 10.5202) (-39.2173, 10.8563) (-39.8314, 11.3105) (-40.5118, 11.9156) knots 0 0 0 0 1 1 1 1
  arc A138 (-40.3043, 12.5997) -> (-40.5118, 11.9156) centre (0, 0) ccw
  spline S138 degree 3 poles (-40.3043, 12.5997) (-39.4023, 12.7248) (-38.6394, 12.7612) (-38.022, 12.753) knots 0 0 0 0 1 1 1 1
  spline S139 degree 3 poles (-38.022, 12.753) (-37.8571, 12.7508) (-37.7028, 12.7454) (-37.5591, 12.7377) knots 0 0 0 0 1 1 1 1
  arc A139 (-37.5591, 12.7377) -> (-37.16, 13.005) centre (-37.5376, 13.1371) ccw
  arc A140 (-36.9754, 13.5211) -> (-37.16, 13.005) centre (0, 0) ccw
  arc A141 (-36.9754, 13.5211) -> (-37.1143, 13.9809) centre (-37.351, 13.6585) ccw
  spline S140 degree 3 poles (-37.1143, 13.9809) (-37.2303, 14.0661) (-37.353, 14.1598) (-37.4818, 14.2627) knots 0 0 0 0 1 1 1 1
  spline S141 degree 3 poles (-37.4818, 14.2627) (-37.9643, 14.648) (-38.531, 15.1601) (-39.1488, 15.8291) knots 0 0 0 0 1 1 1 1
  arc A142 (-38.8752, 16.4895) -> (-39.1488, 15.8291) centre (0, 0) ccw
  spline S142 degree 3 poles (-38.8752, 16.4895) (-37.9653, 16.5257) (-37.2025, 16.4871) (-36.5889, 16.4184) knots 0 0 0 0 1 1 1 1
  spline S143 degree 3 poles (-36.5889, 16.4184) (-36.425, 16.4) (-36.272, 16.3796) (-36.1297, 16.3578) knots 0 0 0 0 1 1 1 1
  arc A143 (-36.1297, 16.3578) -> (-35.7064, 16.5847) centre (-36.0692, 16.7532) ccw
  arc A144 (-35.472, 17.0802) -> (-35.7064, 16.5847) centre (0, 0) ccw
  arc A145 (-35.472, 17.0802) -> (-35.5652, 17.5514) centre (-35.8324, 17.2537) ccw
  spline S144 degree 3 poles (-35.5652, 17.5514) (-35.6723, 17.6475) (-35.7852, 17.7528) (-35.9033, 17.8679) knots 0 0 0 0 1 1 1 1
  spline S145 degree 3 poles (-35.9033, 17.8679) (-36.3458, 18.2986) (-36.8595, 18.8638) (-37.4087, 19.5901) knots 0 0 0 0 1 1 1 1
  arc A146 (-37.0718, 20.2205) -> (-37.4087, 19.5901) centre (0, 0) ccw
  spline S146 degree 3 poles (-37.0718, 20.2205) (-36.1627, 20.1673) (-35.4074, 20.0542) (-34.8034, 19.9257) knots 0 0 0 0 1 1 1 1
  spline S147 degree 3 poles (-34.8034, 19.9257) (-34.6421, 19.8914) (-34.4918, 19.856) (-34.3524, 19.8203) knots 0 0 0 0 1 1 1 1
  arc A147 (-34.3524, 19.8203) -> (-33.9089, 20.0046) centre (-34.2534, 20.2079) ccw
  arc A148 (-33.6271, 20.4748) -> (-33.9089, 20.0046) centre (0, 0) ccw
  arc A149 (-33.6271, 20.4748) -> (-33.6736, 20.9528) centre (-33.9687, 20.6829) ccw
  spline S148 degree 3 poles (-33.6736, 20.9528) (-33.7707, 21.0591) (-33.8728, 21.1749) (-33.9791, 21.301) knots 0 0 0 0 1 1 1 1
  spline S149 degree 3 poles (-33.9791, 21.301) (-34.3772, 21.773) (-34.833, 22.3859) (-35.3084, 23.1625) knots 0 0 0 0 1 1 1 1
  arc A150 (-34.9113, 23.7568) -> (-35.3084, 23.1625) centre (0, 0) ccw
  spline S150 degree 3 poles (-34.9113, 23.7568) (-34.0119, 23.6148) (-33.2712, 23.4282) (-32.6828, 23.2411) knots 0 0 0 0 1 1 1 1
  spline S151 degree 3 poles (-32.6828, 23.2411) (-32.5256, 23.1911) (-32.3795, 23.1411) (-32.2442, 23.092) knots 0 0 0 0 1 1 1 1
  arc A151 (-32.2442, 23.092) -> (-31.7848, 23.232) centre (-32.1077, 23.468) ccw
  arc A152 (-31.4583, 23.6723) -> (-31.7848, 23.232) centre (0, 0) ccw
  arc A153 (-31.4583, 23.6723) -> (-31.4577, 24.1525) centre (-31.7779, 23.9128) ccw
  spline S152 degree 3 poles (-31.4577, 24.1525) (-31.544, 24.2678) (-31.6342, 24.3931) (-31.7276, 24.529) knots 0 0 0 0 1 1 1 1
  spline S153 degree 3 poles (-31.7276, 24.529) (-32.0775, 25.0377) (-32.4711, 25.6923) (-32.8681, 26.5118) knots 0 0 0 0 1 1 1 1
  arc A154 (-32.4146, 27.0644) -> (-32.8681, 26.5118) centre (0, 0) ccw
  spline S154 degree 3 poles (-32.4146, 27.0644) (-31.5334, 26.8348) (-30.8146, 26.5765) (-30.2474, 26.3326) knots 0 0 0 0 1 1 1 1
  spline S155 degree 3 poles (-30.2474, 26.3326) (-30.0959, 26.2675) (-29.9554, 26.2035) (-29.8255, 26.1413) knots 0 0 0 0 1 1 1 1
  arc A155 (-29.8255, 26.1413) -> (-29.3546, 26.2356) centre (-29.6529, 26.5021) ccw
  arc A156 (-28.9865, 26.6417) -> (-29.3546, 26.2356) centre (0, 0) ccw
  arc A157 (-28.9865, 26.6417) -> (-28.9389, 27.1196) centre (-29.281, 26.9124) ccw
  spline S156 degree 3 poles (-28.9389, 27.1196) (-29.0134, 27.2428) (-29.0909, 27.3763) (-29.1706, 27.5207) knots 0 0 0 0 1 1 1 1
  spline S157 degree 3 poles (-29.1706, 27.5207) (-29.4689, 28.0613) (-29.7964, 28.7513) (-30.1112, 29.6058) knots 0 0 0 0 1 1 1 1
  arc A158 (-29.6058, 30.1112) -> (-30.1112, 29.6058) centre (0, 0) ccw
  spline S158 degree 3 poles (-29.6058, 30.1112) (-28.7513, 29.7964) (-28.0613, 29.4689) (-27.5207, 29.1706) knots 0 0 0 0 1 1 1 1
  spline S159 degree 3 poles (-27.5207, 29.1706) (-27.3763, 29.0909) (-27.2428, 29.0134) (-27.1196, 28.9389) knots 0 0 0 0 1 1 1 1
  arc A159 (-27.1196, 28.9389) -> (-26.6417, 28.9865) centre (-26.9124, 29.281) ccw
  arc A160 (-26.2356, 29.3546) -> (-26.6417, 28.9865) centre (0, 0) ccw
  arc A161 (-26.2356, 29.3546) -> (-26.1413, 29.8255) centre (-26.5021, 29.6529) ccw
  spline S160 degree 3 poles (-26.1413, 29.8255) (-26.2035, 29.9554) (-26.2675, 30.0959) (-26.3326, 30.2474) knots 0 0 0 0 1 1 1 1
  spline S161 degree 3 poles (-26.3326, 30.2474) (-26.5765, 30.8146) (-26.8348, 31.5334) (-27.0644, 32.4146) knots 0 0 0 0 1 1 1 1
  arc A162 (-26.5118, 32.8681) -> (-27.0644, 32.4146) centre (0, 0) ccw
  spline S162 degree 3 poles (-26.5118, 32.8681) (-25.6923, 32.4711) (-25.0377, 32.0775) (-24.529, 31.7276) knots 0 0 0 0 1 1 1 1
  spline S163 degree 3 poles (-24.529, 31.7276) (-24.3931, 31.6342) (-24.2678, 31.544) (-24.1525, 31.4577) knots 0 0 0 0 1 1 1 1
  arc A163 (-24.1525, 31.4577) -> (-23.6723, 31.4583) centre (-23.9128, 31.7779) ccw
  arc A164 (-23.232, 31.7848) -> (-23.6723, 31.4583) centre (0, 0) ccw
  arc A165 (-23.232, 31.7848) -> (-23.092, 32.2442) centre (-23.468, 32.1077) ccw
  spline S164 degree 3 poles (-23.092, 32.2442) (-23.1411, 32.3795) (-23.1911, 32.5256) (-23.2411, 32.6828) knots 0 0 0 0 1 1 1 1
  spline S165 degree 3 poles (-23.2411, 32.6828) (-23.4282, 33.2712) (-23.6148, 34.0119) (-23.7568, 34.9113) knots 0 0 0 0 1 1 1 1
  arc A166 (-23.1625, 35.3084) -> (-23.7568, 34.9113) centre (0, 0) ccw
  spline S166 degree 3 poles (-23.1625, 35.3084) (-22.3859, 34.833) (-21.773, 34.3772) (-21.301, 33.9791) knots 0 0 0 0 1 1 1 1
  spline S167 degree 3 poles (-21.301, 33.9791) (-21.1749, 33.8728) (-21.0591, 33.7707) (-20.9528, 33.6736) knots 0 0 0 0 1 1 1 1
  arc A167 (-20.9528, 33.6736) -> (-20.4748, 33.6271) centre (-20.6829, 33.9687) ccw
  arc A168 (-20.0046, 33.9089) -> (-20.4748, 33.6271) centre (0, 0) ccw
  arc A169 (-20.0046, 33.9089) -> (-19.8203, 34.3524) centre (-20.2079, 34.2534) ccw